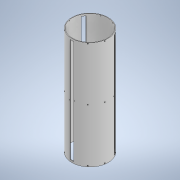
# Autodesk Inventor part: can_closed
Saved by Autodesk Inventor 2021 (Build 250183000, 183)
## iProperties
Created: 2020-09-04
Part Number: can_closed
Material: Generic
Document SubType Name: Modeling
Designer: dsouthall
Density: 1 g/cm^3
Appearance: Default
Author: dsouthall
Autodesk Inventor part; units mm, degrees
sketch "Sketch1" plane through (0, 0, 0) normal (0, 1, 0) x (-1, 0, 0)
  circle A0 centre (0, 0) radius 101.6
  circle A1 centre (0, 0) radius 98.425
  line L0 (0, 98.425) -> (0, -98.425) construction
  line L1 (0, 0) -> (12.080237, 97.68085) construction
  line L2 (0, 0) -> (-12.080237, 97.68085) construction
  line L3 (0, 0) -> (68.66702, 68.66702) construction
  line L4 (0, 0) -> (87.988181, 50.8) construction
  line L5 (0, 0) -> (65.307221, 77.830115) construction
  line L6 (0, 0) -> (100.056468, 17.642655) construction
  line L7 (0, 0) -> (58.144542, 100.709301) construction
  line L8 (0, 0) -> (114.347755, 66.018707) construction
  line L9 (0, 0) -> (-35.703698, 133.248014) construction
  line L10 (0, 0) -> (33.629863, 125.508358) construction
  point P0 (71.842049, 71.842049)
  dimension "OD" = 203.2
  dimension "thickness" = 3.175
  dimension "d13" = 7.05
  dimension "d15" = 7.05
  dimension "end_cap_offset" = 45
  dimension "d75" = 60
  dimension "d88" = 40
  dimension "d89" = 40
  dimension "d90" = 0
  dimension "d91" = 0
  dimension "d119" = 0
  dimension "d120" = 30
  dimension "d121" = 30
  dimension "d147" = 15
  dimension "d148" = 15
  constraints: 22 end point, 8 point on circle, 2 centre point, 1 coincident, 1 point on line, 1 vertical
  measures "OD" diameter of A0
  measures "thickness" radial gap between concentric circles of A1 A0
  measures "d13" angle of L1 L0
  measures "d15" angle of L0 L2
  measures "end_cap_offset" angle of L0 L3
  measures "d75" angle of L4 L0
  measures "d88" angle of L5 L0
  measures "d89" angle of L6 L5
  measures "d90" distance of A0.centre point (0, 0)
  measures "d91" distance of point (0, 0) A0.centre
  measures "d119" distance from line of point (0, 0) L0
  measures "d120" angle of L7 L0
  measures "d121" angle of L8 L7
  measures "d147" angle of L10 L0
  measures "d148" angle of L0 L9
extrude "Extrusion1" add sketch "Sketch1" along normal blind 600
ref_plane "Work Plane1" through (0, 0, 101.6) normal (0, 0, 1) x (1, 0, 0)
sketch "Sketch2" plane through (0, 0, 101.6) normal (0, 0, 1) x (1, 0, 0)
  line L0 (-10, 590) -> (10, 590)
  line L1 (10, 590) -> (10, 10)
  line L2 (10, 10) -> (-10, 10)
  line L3 (-10, 10) -> (-10, 590)
  line L4 (101.6, 600) -> (-101.6, 600) projected
  line L5 (101.6, 0) -> (-101.6, 0) projected
  point P0 (0, 0)
  point P1 (0, 0)
  dimension "edge_height" = 10
  dimension "d5" = 10
  dimension "slot_width" = 20
  dimension "d7" = 10
  constraints: 8 end point, 2 parallel, 1 horizontal, 1 midpoint, 1 perpendicular
  measures "edge_height" distance between parallel lines of L4 L0
  measures "d5" distance between parallel lines of L5 L2
  measures "slot_width" distance between parallel lines of L1 L3
  measures "d7" distance from line of point (0, 0) L1
extrude "Extrusion2" cut sketch "Sketch2" against normal blind 12.7
pattern_circular "Circular Pattern1" count 3 over 360 about axis through (0, 0, 0) along (0, 1, 0) of "Extrusion2"
ref_plane "Central Plane" through (0, 300, 0) normal (0, -1, 0) x (1, 0, 0)
ref_plane "Offset Plane A" through (0, 296.002659, 0) normal (0, -1, 0) x (1, 0, 0)
ref_plane "Offset Plane B" through (0, 303.997341, 0) normal (0, -1, 0) x (1, 0, 0)
ref_plane "Work Plane5" through (-12.469922, 296.002659, 100.831845) normal (-0.1227355, 0, 0.9924394) x (0, -1, 0)
ref_plane "Work Plane6" through (12.469922, 303.997341, 100.831845) normal (0.1227355, 0, 0.9924394) x (0, 1, 0)
hole "Hole1" at (12.469922, 303.997341, 100.831845) direction (-0.1227355, 0, -0.9924394) diameter 2.4384 depth 25.4 countersink diameter 4.699 countersink angle 82 clearance for "Flat Head Machine Screw (82)" size "#2" standard "Ansi Unified Screw Threads"
hole "Hole2" at (-12.469922, 296.002659, 100.831845) direction (0.1227355, 0, -0.9924394) diameter 2.4384 depth 25.4 tip angle 118 countersink diameter 4.699 countersink angle 82 clearance for "Flat Head Machine Screw (82)" size "#2" standard "Ansi Unified Screw Threads"
pattern_circular "Circular Pattern3" count 3 over 360 about axis through (0, 600, 0) along (0, -1, 0) of "Hole1", "Hole2"
ref_plane "Work Plane7" through (-71.842049, 0, 71.842049) normal (-0.7071068, 0, 0.7071068) x (0, -1, 0)
sketch "Sketch6" plane through (-71.842049, 0, 71.842049) normal (-0.7071068, 0, 0.7071068) x (0, -1, 0)
  line L0 (0, 101.6) -> (0, -101.6) construction
  circle A0 centre (0, 0) radius 4.826 construction
  line L1 (-600, 101.6) -> (-600, -101.6) projected
  point P0 (0, 0)
  point P1 (-4.826, 0)
  point P2 (-595.174, 0)
  dimension "d51" = 9.652
  dimension "d64" = 4.826
  constraints: 1 horizontal alignment, 1 midpoint, 2 other
  measures "d64" distance from line of point (-595.174, 0) L1
hole "Hole3" [suppressed]
hole "Hole4" [suppressed]
pattern_circular "Circular Pattern5" [suppressed]
ref_plane "Work Plane12" through (-87.988181, 300, 50.8) normal (-0.8660254, 0, 0.5) x (0, -1, 0)
hole "Hole5" [suppressed]
pattern_circular "Circular Pattern6" [suppressed]
ref_plane "plane for insert hole 1" through (-65.307221, 0, 77.830115) normal (-0.6427876, 0, 0.7660444) x (0, -1, 0)
sketch "Sketch7" plane through (-65.307221, 0, 77.830115) normal (-0.6427876, 0, 0.7660444) x (0, -1, 0)
  point P0 (0, 0)
  point P1 (-300, 0)
  point P2 (-5, 0)
  point P3 (-595, 0)
  dimension "d92" = 0
  dimension "d93" = 300
  dimension "d181" = 0
  dimension "d182" = 0
  dimension "d183" = 295
  dimension "d184" = 295
  measures "d92" vertical distance of point (0, 0) point (-300, 0)
  measures "d93" distance of point (0, 0) point (-300, 0)
  measures "d181" vertical distance of point (-5, 0) point (-300, 0)
  measures "d182" vertical distance of point (-300, 0) point (-595, 0)
  measures "d183" distance of point (-300, 0) point (-5, 0)
  measures "d184" distance of point (-595, 0) point (-300, 0)
ref_plane "plane for insert hole 2" through (-100.056468, 0, 17.642655) normal (-0.9848078, 0, 0.1736482) x (0, -1, 0)
sketch "Sketch8" plane through (-100.056468, 0, 17.642655) normal (-0.9848078, 0, 0.1736482) x (0, -1, 0)
  point P0 (0, 0)
  point P1 (-300, 0)
  point P2 (-5, 0)
  point P3 (-595, 0)
  dimension "d94" = 0
  dimension "d95" = 300
  dimension "d177" = 0
  dimension "d178" = 0
  dimension "d179" = 295
  dimension "d180" = 295
  measures "d94" vertical distance of point (0, 0) point (-300, 0)
  measures "d95" distance of point (0, 0) point (-300, 0)
  measures "d177" vertical distance of point (-300, 0) point (-5, 0)
  measures "d178" vertical distance of point (-300, 0) point (-595, 0)
  measures "d179" distance of point (-300, 0) point (-5, 0)
  measures "d180" distance of point (-595, 0) point (-300, 0)
hole "insert hole 2" at (-100.056468, 300, 17.642655) direction (0.9848078, 0, -0.1736482) diameter 3.2766 depth 8.8646 tip angle 118 countersink diameter 5.715 countersink angle 82 clearance for "Flat Head Machine Screw (82)" size "#4" standard "Ansi Unified Screw Threads"
hole "insert hole 1" at (-65.307221, 300, 77.830115) direction (0.6427876, 0, -0.7660444) diameter 3.2766 depth 8.8646 tip angle 118 countersink diameter 5.715 countersink angle 82 clearance for "Flat Head Machine Screw (82)" size "#4" standard "Ansi Unified Screw Threads"
pattern_circular "Circular Pattern7" count 3 over 360 about axis through (0, 0, 0) along (0, 1, 0) of "insert hole 2"
pattern_circular "Circular Pattern9" count 3 over 360 about axis through (0, 0, 0) along (0, 1, 0) of "insert hole 1"
ref_plane "cap hardware plane 1" through (26.296015, 0, 98.138064) normal (0.258819, 0, 0.9659258) x (0, 1, 0)
ref_plane "cap hardware plane 2" through (-26.296015, 0, 98.138064) normal (-0.258819, 0, 0.9659258) x (0, -1, 0)
sketch "Sketch9" plane through (26.296015, 0, 98.138064) normal (0.258819, 0, 0.9659258) x (0, 1, 0)
  point P0 (0, 0)
  point P1 (5, 0)
  point P2 (595, 0)
  dimension "d149" = 0
  dimension "d150" = 0
  dimension "d151" = 5
  dimension "d152" = 595
  measures "d149" vertical distance of point (0, 0) point (595, 0)
  measures "d150" vertical distance of point (0, 0) point (5, 0)
  measures "d151" distance of point (0, 0) point (5, 0)
  measures "d152" distance of point (0, 0) point (595, 0)
sketch "Sketch10" plane through (-26.296015, 0, 98.138064) normal (-0.258819, 0, 0.9659258) x (0, -1, 0)
  point P0 (0, 0)
  point P1 (-5, 0)
  point P2 (-595, 0)
  dimension "d126" = 0
  dimension "d127" = 0
  dimension "d128" = 5
  dimension "d129" = 595
  measures "d126" vertical distance of point (0, 0) point (-5, 0)
  measures "d127" vertical distance of point (0, 0) point (-595, 0)
  measures "d128" distance of point (0, 0) point (-5, 0)
  measures "d129" distance of point (0, 0) point (-595, 0)
hole "Quad Symmetry Holes 1" [suppressed]
hole "Quad Symmetry Holes 2" [suppressed]
pattern_circular "Circular Pattern11" [suppressed]
hole "Hole13" at (-100.056468, 5, 17.642655) at (-100.056468, 595, 17.642655) direction (0.9848078, 0, -0.1736482) diameter 3.2766 depth 8.8646 tip angle 118 countersink diameter 5.715 countersink angle 82 clearance for "Flat Head Machine Screw (82)" size "#4" standard "Ansi Unified Screw Threads"
hole "Hole14" at (-65.307221, 595, 77.830115) at (-65.307221, 5, 77.830115) direction (0.6427876, 0, -0.7660444) diameter 3.2766 depth 8.8646 tip angle 118 countersink diameter 5.715 countersink angle 82 clearance for "Flat Head Machine Screw (82)" size "#4" standard "Ansi Unified Screw Threads"
pattern_circular "Circular Pattern12" count 3 over 360 about axis through (0, 600, 0) along (0, -1, 0) of "Hole13", "Hole14"
equation "\"d15\" = d13"
equation "\"d5\" = edge_height"
equation "\"d7\" = 0.5 * slot_width"
equation "\"d93\" = 0.5 * height"
equation "\"d184\" = d183"
equation "\"d95\" = 0.5 * height"
equation "\"d180\" = d179"
equation "\"d128\" = d124"
equation "\"d129\" = d125"
equation "\"height\" = 600"
equation "\"d124\" = 5"
equation "\"d125\" = 595"
body "Solid1"
